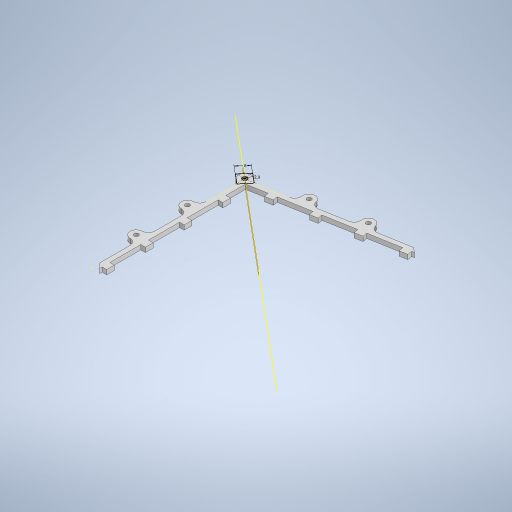
# Autodesk Inventor part: крепежная деталь для клюва
Saved by Autodesk Inventor 2023 (Build 270158000, 158)
## iProperties
Created: 2024-02-14
Part Number: крепежная деталь для клюва
Material: Типовые
Document SubType Name: Modeling
Designer: liza
Density: 1 g/cm^3
Appearance: По умолчанию
Author: liza
Autodesk Inventor part; units mm, degrees
ref_plane "YZ Plane" through (0, 0, 0) normal (1, 0, 0) x (0, 1, 0)
ref_plane "XZ Plane" through (0, 0, 0) normal (0, 1, 0) x (-1, 0, 0)
ref_plane "XY Plane" through (0, 0, 0) normal (0, 0, 1) x (1, 0, 0)
sketch "Эскиз1" plane through (0, 0, 0) normal (1, 0, 0) x (0, 1, 0)
  line L0 (0, 0) -> (3, 0)
  line L1 (3, 0) -> (3, -100)
  line L2 (3, -100) -> (0, -100)
  line L3 (0, -100) -> (0, 0)
  dimension "d0" = 100
  dimension "d2" = 3
  constraints: 8 end point, 2 parallel, 1 horizontal, 1 perpendicular
  measures "d0" distance of L0.end L1.end
  measures "d2" distance of L1.end L2.end
extrude "Выдавливание1" add sketch "Эскиз1" along normal blind 3
sketch "Эскиз2" plane through (3, 0, 0) normal (1, 0, 0) x (0, 0, -1)
  line L0 (4.09, 3) -> (9.09, 3)
  line L1 (9.09, 3) -> (9.09, 0)
  line L2 (9.09, 0) -> (4.09, 0)
  line L3 (4.09, 0) -> (4.09, 3)
  line L4 (100, 3) -> (0, 3) projected
  line L5 (3.7261, 3) -> (3.7261, 3)
  line L6 (6.59, 0) -> (6.59, 0)
  line L7 (0, 0) -> (100, 0) projected
  line L8 (0, 3) -> (0, 0) projected
  dimension "d5" = 5
  dimension "d6" = 3
  dimension "d12" = 4.09
  constraints: 12 end point, 4 parallel, 3 point on line, 2 perpendicular, 1 horizontal, 1 midpoint
  measures "d5" distance of L0.start L0.end
  measures "d6" distance of L0.end L1.end
  measures "d12" distance between parallel lines of L8 L3
extrude "Выдавливание2" add sketch "Эскиз2" along normal blind 3 contours L0 L1 L2 L3
pattern_linear "Прямоуг.массив1" count 4 spacing 25.2 along (0, 0, -1) of "Выдавливание2"
sketch "Эскиз3" plane through (0, 3, 0) normal (0, 1, 0) x (1, 0, 0)
  line L0 (0, 100) -> (0, 0) construction
  line L1 (0, 29.3333) -> (0, 37.3333)
  line L2 (0, 37.3333) -> (-8, 37.3333)
  line L3 (-8, 37.3333) -> (-8, 29.3333)
  line L4 (-8, 29.3333) -> (0, 29.3333)
  circle A0 centre (-4, 33.3333) radius 1.45
  line L5 (-8, 29.3333) -> (0, 37.3333) construction
  line L6 (0, 0) -> (-35.0578, 0) construction
  line L7 (-35.0578, 0) -> (-35.0578, 33.3333) construction
  line L8 (-35.0578, 33.3333) -> (-35.0578, 66.6667) construction
  line L9 (-35.0578, 66.6667) -> (-35.0578, 100) construction
  line L10 (-35.0578, 100) -> (0, 100) construction
  line L11 (-4, 33.3333) -> (-35.0578, 33.3333) construction
  dimension "d13" = 2.9
  dimension "d14" = 8
  dimension "d24" = 33.3333
  constraints: 22 end point, 4 point on line, 3 equal length, 3 perpendicular, 2 horizontal, 2 parallel, 1 centre point, 1 coincident, 1 midpoint
  measures "d13" diameter of A0
  measures "d14" distance of L2.end L3.end
  measures "d24" distance of L7.end L8.end
extrude "Выдавливание3" add sketch "Эскиз3" against normal blind 3
fillet "Сопряжение1" radius 4 4 edges at (0, 1.5, -29.3333) (-8, 1.5, -29.3333) (-8, 1.5, -37.3333) (0, 1.5, -37.3333)
pattern_linear "Прямоуг.массив2" count 2 spacing 33.3333 along (0, 0, -1) of "Сопряжение1", "Выдавливание3"
ref_plane "РабПлоскость1" through (0, 0, -100) normal (-0.6427876, 0, 0.7660444) x (0, 1, 0)
sketch "Эскиз4" plane through (0, 3, 0) normal (0, 1, 0) x (1, 0, 0)
  line L0 (3, 2.4447) -> (0, 5.3135)
  line L1 (0, 5.3135) -> (0, 0)
  line L2 (3, 0) -> (3, 4.09) projected
  line L3 (0, 0) -> (3, 0)
  line L4 (3, 0) -> (3, 2.4447)
  constraints: 8 end point, 1 collinear, 1 perpendicular, 1 vertical
extrude "Выдавливание4" cut sketch "Эскиз4" against normal blind 3
mirror "Зеркальное отражение1" about plane through (0, 0, -100) normal (-0.6427876, 0, 0.7660444)
sketch "Эскиз5" plane through (6, 3, -4.09) normal (0, 1, 0) x (1, 0, 0)
  line L0 (-6, 95.91) -> (-6, 70.5767) construction
  line L1 (-6.9861, 101.959) -> (-12.1284, 95.8307)
  line L2 (-12.1284, 95.8307) -> (-6, 90.6884)
  line L3 (-6, 90.6884) -> (-0.8577, 96.8167)
  line L4 (-0.8577, 96.8167) -> (-6.9861, 101.959)
  line L5 (-6.9861, 101.959) -> (-6, 90.6884) construction
  line L6 (-12.1284, 95.8307) -> (-0.8577, 96.8167) construction
  circle A0 centre (-6.493, 96.3237) radius 1.45
  line L7 (124.1064, -13.2622) -> (-45.1693, 128.777) projected
  line L8 (-6, 95.91) -> (18.9485, 100.3091) construction
  point P0 (-6, -4.09)
  point P1 (-9.5572, 98.8948)
  point P2 (-3.4288, 93.7525)
  dimension "d29" = 2.9
  dimension "d30" = 8
  constraints: 12 end point, 4 midpoint, 3 point on line, 2 parallel, 2 perpendicular, 1 centre point, 1 coincident
  measures "d29" diameter of A0
  measures "d30" distance of L1.start L1.end
extrude "Выдавливание5" add sketch "Эскиз5" against normal blind 3 contours L4 L3 L7 A0 L1 | L7 A0 L3 L2 L1
extrude "Выдавливание6" cut sketch "Эскиз5" against normal blind 3 contours L7 A0 | A0 L7
fillet "Сопряжение2" radius 4 4 edges at (-6.1284, 1.5, -99.9207) (0, 1.5, -94.7784) (-0.9861, 1.5, -106.049) (5.1423, 1.5, -100.9067)
